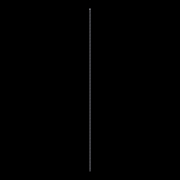
# Autodesk Inventor part: Rod
Saved by Autodesk Inventor 2012 (Build 160160000, 160)
## iProperties
Created: 2012-10-02
Part Number: Rod
Material: Steel, Mild
Document SubType Name: Modeling
Designer: agmlego
Density: 7.86 g/cm^3
Mass: 16.6649 g
Surface Area: 28.3926 cm^2
Volume: 2.12021 cm^3
Author: agmlego
Autodesk Inventor part; units mm, degrees
ref_plane "YZ Plane" through (0, 0, 0) normal (1, 0, 0) x (0, 1, 0)
ref_plane "XZ Plane" through (0, 0, 0) normal (0, 1, 0) x (-1, 0, 0)
ref_plane "XY Plane" through (0, 0, 0) normal (0, 0, 1) x (1, 0, 0)
sketch "Sketch1" plane through (0, 0, 0) normal (0, 0, 1) x (1, 0, 0)
  circle A0 centre (0, 0) radius 1.5
  dimension "d0" = 3
  constraints: 1 centre point, 1 coincident
  measures "d0" diameter of A0
extrude "Extrusion1" add sketch "Sketch1" along normal blind 300
chamfer "Chamfer1" distance 0.2 angle 45 2 edges at (-1.5, 0, 300) (-1.5, 0, 0)
thread "Thread1" size "M3x0.5" class "6g" standard "ANSI Metric M Profile" full length
body "Solid1"
